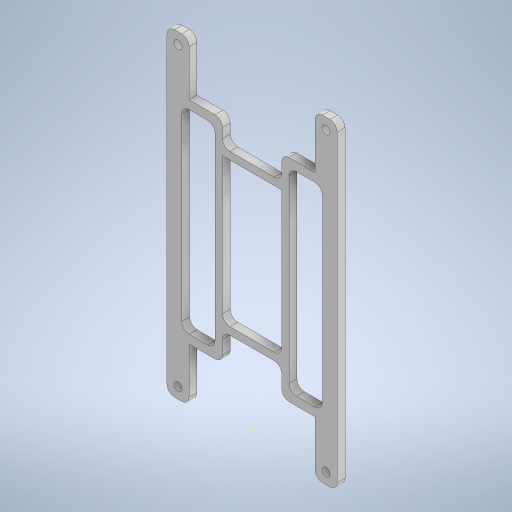
# Autodesk Inventor part: connector_meta_v2l
Saved by Autodesk Inventor 2024 (Build 280153000, 153)
## iProperties
Created: 2023-02-15
Part Number: connector_meta_v2l
Material: Generic
Document SubType Name: Modeling
Designer: pawel
Density: 1 g/cm^3
Appearance: Default
Author: pawel
Autodesk Inventor part; units mm, degrees
ref_plane "YZ Plane" through (0, 0, 0) normal (1, 0, 0) x (0, 1, 0)
ref_plane "XZ Plane" through (0, 0, 0) normal (0, 1, 0) x (-1, 0, 0)
ref_plane "XY Plane" through (0, 0, 0) normal (0, 0, 1) x (1, 0, 0)
sketch "Sketch1" plane through (0, 0, 0) normal (0, 0, 1) x (1, 0, 0)
  circle A0 centre (-20, 0) radius 1.1
  circle A1 centre (20, 0) radius 1.1
  line L0 (-17, 0) -> (-17, -1)
  line L1 (-19, -3) -> (-21, -3)
  line L2 (-23, -1) -> (-23, 2)
  circle A2 centre (-20, 80) radius 1.1
  circle A3 centre (20, 80) radius 1.1
  line L3 (-23, 2) -> (-23, 81)
  line L4 (17, 0) -> (17, -1)
  line L5 (19, -3) -> (21, -3)
  line L6 (23, -1) -> (23, 2)
  line L7 (23, 2) -> (23, 81)
  line L8 (-17, 0) -> (-17, 80)
  line L9 (17, 0) -> (17, 80)
  line L10 (-21, 83) -> (-19, 83)
  line L11 (-17, 81) -> (-17, 80)
  line L12 (21, 83) -> (19, 83)
  line L13 (17, 81) -> (17, 79.5158)
  line L14 (-17, 11.4131) -> (17, 11.4131)
  line L15 (-17, 68.5869) -> (17, 68.5869)
  line L16 (-10, 15.7355) -> (-10, 64.2645)
  line L17 (-8, 15.7355) -> (-8, 64.2645)
  line L18 (10, 15.7355) -> (10, 64.2645)
  line L19 (8, 15.7355) -> (8, 64.2645)
  arc A4 (-21, 83) -> (-23, 81) centre (-21, 81) ccw
  arc A5 (-17, 81) -> (-19, 83) centre (-19, 81) ccw
  arc A6 (19, 83) -> (17, 81) centre (19, 81) ccw
  arc A7 (23, 81) -> (21, 83) centre (21, 81) ccw
  arc A8 (-19, -3) -> (-17, -1) centre (-19, -1) ccw
  arc A9 (-23, -1) -> (-21, -3) centre (-21, -1) ccw
  arc A10 (17, -1) -> (19, -3) centre (19, -1) ccw
  arc A11 (21, -3) -> (23, -1) centre (21, -1) ccw
  line L20 (-12, 13.7355) -> (-17, 13.7355)
  line L21 (17, 13.7355) -> (12, 13.7355)
  line L22 (6, 13.7355) -> (-6, 13.7355)
  line L23 (17, 66.2645) -> (12, 66.2645)
  line L24 (-12, 66.2645) -> (-17, 66.2645)
  line L25 (6, 66.2645) -> (-6, 66.2645)
  arc A12 (-8, 15.7355) -> (-6, 13.7355) centre (-6, 15.7355) ccw
  arc A13 (-12, 13.7355) -> (-10, 15.7355) centre (-12, 15.7355) ccw
  arc A14 (6, 13.7355) -> (8, 15.7355) centre (6, 15.7355) ccw
  arc A15 (10, 15.7355) -> (12, 13.7355) centre (12, 15.7355) ccw
  arc A16 (-6, 66.2645) -> (-8, 64.2645) centre (-6, 64.2645) ccw
  arc A17 (-10, 64.2645) -> (-12, 66.2645) centre (-12, 64.2645) ccw
  arc A18 (8, 64.2645) -> (6, 66.2645) centre (6, 64.2645) ccw
  arc A19 (12, 66.2645) -> (10, 64.2645) centre (12, 64.2645) ccw
  point P0 (17, 83)
  constraints: 52 end point, 32 point on circle, 32 tangent, 20 centre point, 14 equal radius, 10 perpendicular, 8 point on line, 2 vertical, 1 horizontal
extrude "Extrusion1" add sketch "Sketch1" along normal blind 3 contours L0 A8 L1 A9 L2 L3 A4 L10 A5 L11 L8 | L9 L13 A6 L12 A7 L7 L6 A11 L5 A10 L4
extrude "Extrusion2" add sketch "Sketch1" along normal blind 3 contours L8 L20 A13 L16 A17 L24 L15 L9 L23 A19 L18 A15 L21 L14
sketch "Sketch2" plane through (0, 0, 3) normal (0, 0, 1) x (1, 0, 0)
  line L0 (-21, 83) -> (-19, 83)
  line L1 (-17, 81) -> (-17, -1)
  line L2 (-19, -3) -> (-21, -3)
  line L3 (-23, -1) -> (-23, 81)
  line L4 (19, -3) -> (21, -3)
  line L5 (23, -1) -> (23, 81)
  line L6 (21, 83) -> (19, 83)
  line L7 (17, 81) -> (17, -1)
  arc A0 (-21, 83) -> (-23, 81) centre (-21, 81) ccw
  arc A1 (-17, 81) -> (-19, 83) centre (-19, 81) ccw
  arc A2 (-19, -3) -> (-17, -1) centre (-19, -1) ccw
  arc A3 (-23, -1) -> (-21, -3) centre (-21, -1) ccw
  arc A4 (21, -3) -> (23, -1) centre (21, -1) ccw
  arc A5 (17, -1) -> (19, -3) centre (19, -1) ccw
  arc A6 (19, 83) -> (17, 81) centre (19, 81) ccw
  arc A7 (23, 81) -> (21, 83) centre (21, 81) ccw
  circle A8 centre (20, 80) radius 1.1
  circle A9 centre (20, 0) radius 1.1
  circle A10 centre (-20, 0) radius 1.1
  circle A11 centre (-20, 80) radius 1.1007
  point P0 (0, 0)
  point P1 (17, -3)
  dimension "d9" = 2
  constraints: 16 end point, 16 point on circle, 16 tangent, 12 centre point, 7 equal radius, 4 parallel, 3 point on line, 2 horizontal, 2 perpendicular
  measures "d9" radius of A0
extrude "Extrusion3" add sketch "Sketch2" along normal blind 1
sketch "Szkic3" plane through (0, 0, 4) normal (0, 0, 1) x (1, 0, 0)
  line L0 (-65, 108) -> (57, 108)
  line L1 (57, 108) -> (57, -17)
  line L2 (57, -17) -> (-65, -17)
  line L3 (-65, -17) -> (-65, 108)
  point P0 (0, 0)
  constraints: 8 end point, 2 parallel, 1 horizontal, 1 perpendicular
extrude "Wyciągnięcie proste4" cut sketch "Szkic3" against normal blind 2
sketch "Szkic4" plane through (0, 0, 2) normal (0, 0, 1) x (1, 0, 0)
  line L0 (-8, 71) -> (8, 71)
  line L1 (8, 71) -> (8, 3)
  line L2 (8, 3) -> (-8, 3)
  line L3 (-8, 3) -> (-8, 71)
  point P0 (0, 0)
  constraints: 8 end point, 2 parallel, 1 horizontal, 1 perpendicular
extrude "Wyciągnięcie proste5" cut sketch "Szkic4" against normal blind 2
sketch "Szkic5" plane through (0, 0, 2) normal (0, 0, 1) x (1, 0, 0)
  line L0 (-8, 11.4131) -> (-8, 68.5869) projected
  line L1 (8, 68.5869) -> (8, 11.4131) projected
  line L2 (-8, 62) -> (8, 62)
  line L3 (8, 62) -> (8, 19)
  line L4 (8, 19) -> (-8, 19)
  line L5 (-8, 19) -> (-8, 62)
  line L6 (-8, 60) -> (9, 60)
  line L7 (-8, 21) -> (8, 21)
  point P0 (0, 0)
  point P1 (8, 60)
  constraints: 12 end point, 5 point on line, 3 perpendicular, 2 parallel, 1 horizontal
extrude "Wyciągnięcie proste6" add sketch "Szkic5" against normal blind 2 contours L0 L7 L1 L4 | L0 L2 L1 L6
fillet "Zaokrąglenie1" radius 2 10 edges at (-8, 68.5869, 1) (8, 68.5869, 1) (8, 11.4131, 1) (-8, 11.4131, 1) (-8, 19, 1) (8, 19, 1) (8, 21, 1) (-8, 21, 1) (-8, 62, 1) (8, 62, 1)
sketch "Szkic7" plane through (0, 0, 2) normal (0, 0, 1) x (1, 0, 0)
  point P0 (0, 0)
sketch "Szkic8" plane through (0, 0, 2) normal (0, 0, 1) x (1, 0, 0)
  line L0 (-19, 66.2645) -> (19, 66.2645)
  line L1 (19, 66.2645) -> (19, 13.7355)
  line L2 (19, 13.7355) -> (-19, 13.7355)
  line L3 (-19, 13.7355) -> (-19, 66.2645)
  line L4 (-16, 66.2645) -> (-16, 13.7355)
  line L5 (12, 66.2645) -> (17, 66.2645) projected
  line L6 (16, 66.2645) -> (16, 13.7355)
  point P0 (0, 0)
  constraints: 12 end point, 4 point on line, 3 perpendicular, 2 parallel, 1 horizontal
extrude "Wyciągnięcie proste8" cut sketch "Szkic8" against normal blind 10 contours L0 L4 L2 L3 | L0 L1 L2 L6
fillet "Zaokrąglenie2" radius 2 4 edges at (19, 66.2645, 1) (19, 13.7355, 1) (-19, 66.2645, 1) (-19, 13.7355, 1)
thicken "Pogrubienie1" operation add thickness 0.1 both sides no extend neighbours no toward (0, 0, 1) faces at (-21.6667, 31.9118, 2)
body "Solid1"
